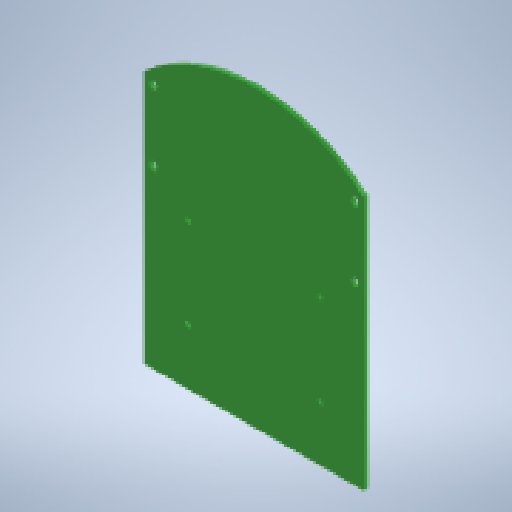
# Autodesk Inventor part: BaseBoard-SPG27
Saved by Autodesk Inventor 2025.3 (Build 293356030, 356C)
## iProperties
Created: 2025-05-29
Part Number: BaseBoard-SPG27
Material: 一般
Document SubType Name: Modeling
Designer: yamashita1
Density: 1 g/cm^3
Appearance: 滑らか - 濃い深緑
Author: yamashita1
Autodesk Inventor part; units mm, degrees
ref_plane "YZ Plane" through (0, 0, 0) normal (1, 0, 0) x (0, 1, 0)
ref_plane "XZ Plane" through (0, 0, 0) normal (0, 1, 0) x (-1, 0, 0)
ref_plane "XY Plane" through (0, 0, 0) normal (0, 0, 1) x (1, 0, 0)
sketch "スケッチ1" plane through (0, 0, 0) normal (0, 0, 1) x (1, 0, 0)
  circle A0 centre (0, 0) radius 65 construction
  line L0 (-42.5, 65) -> (42.5, 65) construction
  line L1 (42.5, 65) -> (42.5, -65) construction
  line L2 (42.5, -65) -> (-42.5, -65) construction
  line L3 (-42.5, -65) -> (-42.5, 65) construction
  arc A1 (42.5, 49.1808) -> (-42.5, 49.1808) centre (0, 0) ccw
  line L4 (-42.5, 49.1808) -> (-42.5, -49.1808)
  line L5 (42.5, 49.1808) -> (42.5, -49.1808)
  arc A2 (-42.5, -49.1808) -> (42.5, -49.1808) centre (0, 0) ccw
  line L6 (42.5, -49) -> (-42.5, -49)
  point P0 (0, 65)
  dimension "d0" = 130
  dimension "d1" = 85
  dimension "d41" = 49
  constraints: 16 end point, 9 point on circle, 6 point on line, 3 centre point, 3 parallel, 2 perpendicular, 2 tangent, 1 coincident, 1 concentric, 1 horizontal, 1 midpoint, 1 vertical, 1 vertical alignment
  measures "d0" diameter of A0
  measures "d1" distance of L1.end L2.end
  measures "d41" distance from line of point (0, 0) L6
extrude "基板" add sketch "スケッチ1" along normal blind 1.6 contours L5 L6 L4 A1
sketch "スケッチ2" plane through (0, 0, 1.6) normal (0, 0, 1) x (1, 0, 0)
  line L0 (0, 110.7931) -> (0, -110.7931) construction
  line L1 (-42.5, 49.1808) -> (-42.5, -49) construction
  line L2 (-63.4163, -10) -> (63.4163, -10) construction
  point P0 (0, 0)
  point P1 (0, 0)
  point P2 (0, 0)
  point P3 (-42.5, -49.1808)
  point P4 (-25.5, -27.5)
  point P5 (-25.5, 7.5)
  point P6 (25.5, -27.5)
  point P7 (25.5, 7.5)
  point P8 (0, -10)
  dimension "d38" = 35
  dimension "d39" = 17
  dimension "d40" = 10
  constraints: 4 end point, 2 coincident, 2 horizontal alignment, 2 midpoint, 2 symmetric about line, 1 horizontal, 1 point on line, 1 vertical, 1 vertical alignment
  measures "d38" distance of point (-25.5, 7.5) point (-25.5, -27.5)
  measures "d39" distance from line of L1 point (-25.5, -27.5)
  measures "d40" distance from line of L2 point (0, 0)
hole "モータ取付穴" at (-25.5, -27.5, 1.6) at (-25.5, 7.5, 1.6) at (25.5, -27.5, 1.6) at (25.5, 7.5, 1.6) direction (0, 0, -1) diameter 2.1 end through all
sketch "スケッチ6" plane through (0, 0, 0) normal (0, 0, -1) x (-1, 0, 0)
  line L0 (0, 0) -> (0, 96.2051) construction
  point P0 (39, 46)
  point P1 (-39, 46)
  point P2 (-39, 19)
  point P3 (39, 19)
  dimension "d52" = 78
  dimension "d53" = 27
  dimension "d54" = 46
  constraints: 2 end point, 2 symmetric about line, 1 horizontal alignment, 1 vertical, 1 vertical alignment
  measures "d52" distance of point (-39, 46) point (39, 46)
  measures "d53" distance of point (-39, 19) point (-39, 46)
  measures "d54" vertical distance of L0.start point (39, 46)
hole "連結穴" at (-39, 46, 0) at (39, 46, 0) at (39, 19, 0) at (-39, 19, 0) direction (0, 0, 1) diameter 3.2 end through all
